Tubing Adaptor_v7 (Autodesk Fusion 360 design; units mm, degrees)
Autodesk Fusion 360 part; units mm, degrees
sketch "Sketch1" plane through (0, 0, 0) normal (0, 0, 1) x (1, 0, 0)
  circle A0 centre (0, 0) radius 6
  circle A1 centre (0, 0) radius 4.5
  circle A2 centre (0, 0) radius 8.25
  circle A3 centre (0, 0) radius 9.75
  circle A4 centre (0, 0) radius 5.5
  circle A5 centre (0, 0) radius 11.25
  dimension "d1" = 12
  dimension "d2" = 9
  dimension "d3" = 16.5
  dimension "d4" = 19.5
  dimension "d10" = 11
  dimension "d36" = 22.5
  constraint coincident A0.centre A1.centre
  constraint concentric A2 A3
  constraint concentric A3 A4
  constraint concentric A4 A5
  measures "d1" diameter of A0
  measures "d2" diameter of A1
  measures "d3" diameter of A2
  measures "d4" diameter of A3
  measures "d10" diameter of A4
  measures "d36" diameter of A5
ref_plane "WorkPlane1" through (0, 0, 6) normal (0, 0, 1) x (1, 0, 0)
sketch "Sketch2" plane through (0, 0, 6) normal (0, 0, 1) x (1, 0, 0)
  circle A0 centre (0, 0) radius 4.5
  circle A1 centre (0, 0) radius 5.5
  dimension "d6" = 9
  dimension "d7" = 11
  constraint coincident A0.centre A1.centre
  constraint concentric A0 A1
  measures "d6" diameter of A0
  measures "d7" diameter of A1
loft "Loft1" add profiles "Sketch1", "Sketch2" section 1 contours A0 | A4 section 2
extrude "Extrude1" cut sketch "Sketch2" against normal blind 6 contours A0
extrude "Extrude2" add sketch "Sketch1" against normal blind 14 contours A4
extrude "Extrude3" add sketch "Sketch1" against normal blind 2 from surface at -12 contours A0 | A2 | A3 | A5
sketch "Sketch3" plane through (0, 0, -14) normal (0, 0, -1) x (1, 0, 0)
  circle A0 centre (0, 0) radius 4.5
  circle A1 centre (0, 0) radius 6
  circle A2 centre (0, 0) radius 8.1
  circle A3 centre (0, 0) radius 10
  circle A4 centre (0, 0) radius 10
  circle A5 centre (0, 0) radius 11.25
  circle A6 centre (0, 0) radius 7.9
  circle A7 centre (0, 0) radius 11.25
  dimension "d18" = 12
  dimension "d21" = 16.2
  dimension "d22" = 22.5
  dimension "d25" = 15.8
  constraint concentric A1 A2
  constraint concentric A2 A3
  constraint concentric A3 A4
  constraint concentric A2 A5
  constraint concentric A4 A6
  measures "d18" diameter of A1
  measures "d21" diameter of A2
  measures "d22" diameter of A5
  measures "d25" diameter of A6
extrude "Extrude5" add sketch "Sketch3" along normal blind 10 contours A1
extrude "Extrude6" add sketch "Sketch3" along normal blind 10 contours A3 A4 | A5 A7
extrude "Extrude7" add sketch "Sketch3" along normal blind 0.5 from surface at 4.75 contours A2
chamfer "Chamfer3" distance 0.2 angle 45 1 edges at (-7.5519, 2.9291, -18.75) measured on face at (8.0597, 0.8065, -15.5833)
chamfer "Chamfer4" distance 0.2 angle 45 1 edges at (-7.5519, -2.9291, -19.25) measured on face at (8.0597, 0.8065, -20.8333)
sketch "Sketch5" plane through (0, 0, -24) normal (0, 0, -1) x (1, 0, 0)
  circle A0 centre (0, 0) radius 11.25
  circle A1 centre (0, 0) radius 8.1
  line L0 (-9, 1) -> (9, 1)
  line L1 (9, 1) -> (9, -1)
  line L2 (9, -1) -> (-9, -1)
  line L3 (-9, -1) -> (-9, 1)
  line L4 (-1, 10) -> (1, 10)
  line L5 (1, 10) -> (1, -10)
  line L6 (1, -10) -> (-1, -10)
  line L7 (-1, -10) -> (-1, 10)
  circle A2 centre (0, 0) radius 4.5
  circle A3 centre (0, 0) radius 6
  constraint horizontal L0
  constraint vertical L1
  constraint horizontal L2
  constraint vertical L3
  constraint horizontal L4
  constraint vertical L5
  constraint horizontal L6
  constraint vertical L7
extrude "Extrude10" add sketch "Sketch5" against normal blind 1 contours A1 L0 L2 A3 | A1 L5 L7 A3 | A1 L5 L7 A3 | A1 L0 L2 A3
chamfer "Chamfer7" distance 0.5 angle 45 1 edges at (-5.1278, -1.9889, 0) measured on face at (5.811, -0.2981, 0)
chamfer "Chamfer8" distance 1 angle 45 1 edges at (-5.1278, -1.9889, -12) measured on face at (5.4727, -0.5476, -4.3333)
